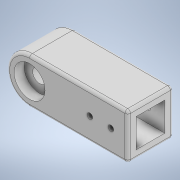
# Autodesk Inventor part: băng chuyền
Saved by Autodesk Inventor 2020 (Build 240168000, 168)
## iProperties
Created: 2022-11-30
Part Number: băng chuyền
Material: Generic
Document SubType Name: Modeling
Designer: ADMIN
Density: 1 g/cm^3
Appearance: Default
Author: ADMIN
Autodesk Inventor part; units mm, degrees
ref_plane "YZ Plane" through (0, 0, 0) normal (1, 0, 0) x (0, 1, 0)
ref_plane "XZ Plane" through (0, 0, 0) normal (0, 1, 0) x (-1, 0, 0)
ref_plane "XY Plane" through (0, 0, 0) normal (0, 0, 1) x (1, 0, 0)
sketch "Sketch1" plane through (0, 0, 0) normal (0, 0, 1) x (1, 0, 0)
  line L0 (16.2, 0) -> (86.2, 0)
  line L1 (86.2, 0) -> (86.2, -32.4)
  line L2 (86.2, -32.4) -> (16.2, -32.4)
  circle A0 centre (16.2, -16.2) radius 5
  circle A1 centre (59.2, -16.2) radius 2
  circle A2 centre (74.2, -16.2) radius 2
  arc A3 (16.2, 0) -> (16.2, -32.4) centre (16.2, -16.2) ccw
  point P0 (0, 0)
  dimension "d1" = 32.4
  dimension "d2" = 10
  dimension "d4" = 16.2
  dimension "d5" = 4
  dimension "d6" = 43
  dimension "d7" = 4
  dimension "d8" = 15
  dimension "d9" = 32.4
  constraints: 6 end point, 4 centre point, 2 point on circle, 1 coincident, 1 horizontal, 1 parallel, 1 perpendicular
  measures "d1" distance of L0.end L1.end
  measures "d2" diameter of A0
  measures "d4" distance from line of L0 A0.centre
  measures "d5" diameter of A1
  measures "d6" distance of A0.centre A1.centre
  measures "d7" diameter of A2
  measures "d8" distance of A1.centre A2.centre
  measures "d9" diameter of A3
extrude "Extrusion1" add sketch "Sketch1" along normal blind 32.4
sketch "Sketch2" plane through (86.2, -32.4, 0) normal (1, 0, 0) x (0, 0, -1)
  line L0 (0, 32.4) -> (-32.4, 32.4) projected
  line L1 (0, 0) -> (0, 32.4) projected
  line L2 (-26.45, 5.95) -> (-5.95, 5.95)
  line L3 (-5.95, 5.95) -> (-5.95, 26.45)
  line L4 (-5.95, 26.45) -> (-26.45, 26.45)
  line L5 (-26.45, 26.45) -> (-26.45, 5.95)
  line L6 (-26.45, 5.95) -> (-5.95, 26.45) construction
  line L7 (-5.95, 5.95) -> (-26.45, 26.45) construction
  dimension "d12" = 20.5
  dimension "d13" = 20.5
  constraints: 12 end point, 2 parallel, 1 horizontal, 1 perpendicular
  measures "d12" distance of L4.end L3.end
  measures "d13" distance of L3.end L2.end
extrude "Extrusion2" cut sketch "Sketch2" against normal blind 50
sketch "Sketch3" plane through (0, 0, 32.4) normal (0, 0, 1) x (1, 0, 0)
  circle A0 centre (16.2, -16.2) radius 5 projected
  circle A1 centre (16.2, -16.2) radius 11.03
  point P0 (0, 0)
  dimension "d16" = 22.06
  constraints: 1 centre point, 1 coincident
  measures "d16" diameter of A1
extrude "Extrusion3" cut sketch "Sketch3" against normal blind 7.2
fillet "Fillet1" radius 2 10 edges at (0, -16.2, 32.4) (51.2, -32.4, 32.4) (51.2, 0, 32.4) (0, -16.2, 0) (51.2, -32.4, 0) (51.2, 0, 0) (86.2, 0, 16.2) (86.2, -16.2, 32.4) (86.2, -16.2, 0) (86.2, -32.4, 16.2)
body "Solid1"
